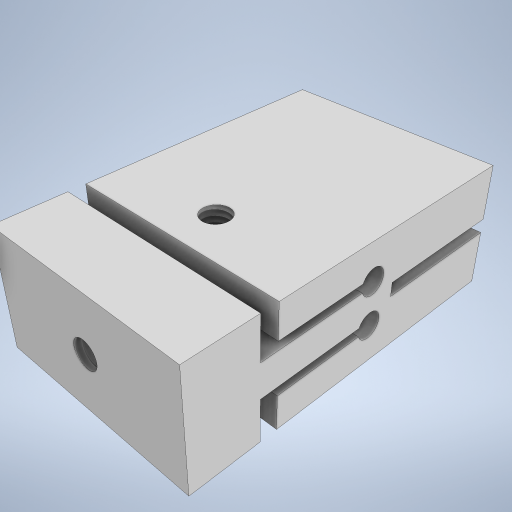
# Autodesk Inventor part: holder_slide_1.5mmThick_25mmWide
Saved by Autodesk Inventor 2023 (Build 270158000, 158)
## iProperties
Created: 2023-09-25
Part Number: holder_slide_1.5mmThick_25mmWide
Material: Generic
Document SubType Name: Modeling
Designer: nvladi
Density: 1 g/cm^3
Appearance: Default
Author: nvladi
Autodesk Inventor part; units mm, degrees
note: some values were not read from the file. Chosen so that the rebuilt part matches the saved one: direction of "Hole2"; direction of "Hole3".
ref_plane "YZ Plane" through (0, 0, 0) normal (1, 0, 0) x (0, 1, 0)
ref_plane "XZ Plane" through (0, 0, 0) normal (0, 1, 0) x (-1, 0, 0)
ref_plane "XY Plane" through (0, 0, 0) normal (0, 0, 1) x (1, 0, 0)
sketch "Sketch1" plane through (0, 0, 0) normal (0, 0, 1) x (1, 0, 0)
  line L0 (12.5, -7) -> (-12.5, -7)
  line L1 (-12.5, -7) -> (-12.5, 7)
  line L2 (-12.5, 7) -> (12.5, 7)
  line L3 (12.5, 7) -> (12.5, -7)
  line L4 (12.5, -7) -> (-12.5, 7) construction
  line L5 (-12.5, -7) -> (12.5, 7) construction
  point P0 (0, 0)
  dimension "d0" = 25
  dimension "d1" = 14
  constraints: 12 end point, 2 midpoint, 2 parallel, 1 horizontal, 1 perpendicular
  measures "d0" distance of L1.end L2.end
  measures "d1" distance of L0.end L1.end
extrude "Extrusion1" add sketch "Sketch1" along normal blind 30
sketch "Sketch2" plane through (0, 0, 0) normal (0, 0, -1) x (-1, 0, 0)
  line L0 (15, -0.8) -> (-15, -0.8)
  line L1 (-15, -0.8) -> (-15, 0.8)
  line L2 (-15, 0.8) -> (15, 0.8)
  line L3 (15, 0.8) -> (15, -0.8)
  line L4 (15, -0.8) -> (-15, 0.8) construction
  line L5 (-15, -0.8) -> (15, 0.8) construction
  point P0 (0, 0)
  dimension "d4" = 30
  dimension "d5" = 1.6
  constraints: 12 end point, 2 midpoint, 2 parallel, 1 horizontal, 1 perpendicular
  measures "d4" distance of L1.end L2.end
  measures "d5" distance of L0.end L1.end
extrude "Extrusion2" cut sketch "Sketch2" against normal blind 15
sketch "Sketch4" plane through (12.5, -7, 30) normal (1, 0, 0) x (0, 0, -1)
  line L0 (-12, 4.5) -> (12, 4.5)
  line L1 (12, 4.5) -> (12, 9.5)
  line L2 (12, 9.5) -> (-12, 9.5)
  line L3 (-12, 9.5) -> (-12, 4.5)
  line L4 (0, 0) -> (0, 14) projected
  line L5 (-12, 4.5) -> (12, 9.5) construction
  line L6 (12, 4.5) -> (-12, 9.5) construction
  line L7 (30, 0) -> (0, 0) projected
  circle A0 centre (12, 9.5) radius 1.5
  circle A1 centre (12, 4.5) radius 1.5
  line L8 (-12, 9) -> (12, 9)
  line L9 (12, 9) -> (12, 10)
  line L10 (12, 10) -> (-12, 10)
  line L11 (-12, 10) -> (-12, 9)
  line L12 (0, 14) -> (0, 0) projected
  line L13 (-12, 9) -> (12, 10) construction
  line L14 (12, 9) -> (-12, 10) construction
  line L15 (-12, 4) -> (12, 4)
  line L16 (12, 4) -> (12, 5)
  line L17 (12, 5) -> (-12, 5)
  line L18 (-12, 5) -> (-12, 4)
  line L19 (-12, 4) -> (12, 5) construction
  line L20 (12, 4) -> (-12, 5) construction
  point P0 (30, 7)
  point P1 (0, 7)
  point P2 (0, 9.5)
  point P3 (0, 4.5)
  point P4 (10.5858, 5)
  point P5 (10.5858, 4)
  point P6 (10.5858, 10)
  point P7 (-12, 9)
  point P8 (10.5858, 9)
  dimension "d16" = 5
  dimension "d17" = 3
  dimension "d18" = 3
  dimension "d19" = 1
  dimension "d20" = 1
  dimension "d23" = 12
  constraints: 36 end point, 9 midpoint, 8 parallel, 4 perpendicular, 2 centre point, 2 coincident, 2 collinear, 2 point on line
  measures "d16" distance of L1.end L0.end
  measures "d17" diameter of A0
  measures "d18" diameter of A1
  measures "d19" distance of L9.end L8.end
  measures "d20" distance of L16.end L15.end
  measures "d23" distance between parallel lines of L4 L1
extrude "Extrusion3" cut sketch "Sketch4" against normal through all contours L3 L17 L4 L0 | L0 L4 L15 L18 | L4 L17 A1 L0 | L0 A1 L15 L4 | A1 L17 L1 L0 | L0 L16 L15 A1 | L3 L2 L4 L8 | L1 A1 L15 L16 | A1 L1 L17 | L4 L2 A0 L8 | L11 L10 L4 L2 | L4 L10 A0 L2 | L8 L1 A0 | A0 L2 L1 L8 | L1 L9 L10 A0 | A0 L10 L9 L2
sketch "Sketch5" plane through (-12.5, 7, 0) normal (0, 1, 0) x (1, 0, 0)
  line L0 (25, -30) -> (0, -30) projected
  point P0 (12.5, 0)
  point P1 (12.5, -25)
  point P2 (12.5, -30)
  dimension "d24" = 5
  constraints: 1 midpoint
  measures "d24" distance of point (12.5, -30) point (12.5, -25)
sketch "Sketch6" plane through (-12.5, -7, 0) normal (0, -1, 0) x (1, 0, 0)
  point P0 (12.5, 0)
  point P1 (12.5, 25)
hole "Hole2" at (0, -7, 25) direction (0, 1, 0) diameter 3.242 depth 4 thread size "M4x0.7" class "6H" standard "ISO Metric profile"
hole "Hole3" at (0, 7, 25) direction (0, -1, 0) diameter 3.242 depth 4 thread size "M4x0.7" class "6H" standard "ISO Metric profile"
sketch "Sketch7" plane through (0, 0, 30) normal (0, 0, 1) x (1, 0, 0)
  line L0 (-12.5, -2) -> (12.5, -2) projected
  line L1 (12.5, -2) -> (12.5, 2) projected
  line L2 (12.5, 2) -> (-12.5, 2) projected
  line L3 (-12.5, 2) -> (-12.5, -2) projected
  point P0 (0, 0)
extrude "Extrusion4" add sketch "Sketch7" along normal blind 2
sketch "Sketch11" plane through (0, 0, 32) normal (0, 0, 1) x (1, 0, 0)
  line L0 (-12.5, 7) -> (-12.5, 0.8) projected
  line L1 (12.5, -7) -> (-12.5, -7)
  line L2 (-12.5, -7) -> (-12.5, 7)
  line L3 (-12.5, 7) -> (12.5, 7)
  line L4 (12.5, 7) -> (12.5, -7)
  line L5 (12.5, -7) -> (-12.5, 7) construction
  line L6 (-12.5, -7) -> (12.5, 7) construction
  point P0 (0, 0)
  point P1 (-12.5, 0.8)
  constraints: 12 end point, 2 midpoint, 2 parallel, 1 horizontal, 1 perpendicular
extrude "Extrusion6" add sketch "Sketch11" along normal blind 8
sketch "Sketch12" plane through (0, 0, 40) normal (0, 0, 1) x (1, 0, 0)
  point P0 (0, 0)
  point P1 (0, 0)
  constraints: 1 coincident
hole "Hole4" at (0, 0, 40) direction (0, 0, -1) diameter 3.242 depth 7 thread size "M4x0.7" class "6H" standard "ISO Metric profile"
body "Solid1"
